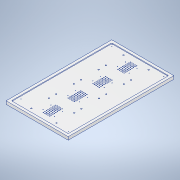
# Autodesk Inventor part: Tamale Assembly Plate
Saved by Autodesk Inventor 2022 (Build 260153000, 153)
## iProperties
Created: 2021-07-29
Part Number: Tamale Assembly Plate
Material: Aluminum 6061
Document SubType Name: Modeling
Designer: Caleb
Density: 2.7 g/cm^3
Appearance: Aluminum - Flat
Author: Caleb
Autodesk Inventor part; units mm, degrees
ref_plane "YZ Plane" through (0, 0, 0) normal (1, 0, 0) x (0, 1, 0)
ref_plane "XZ Plane" through (0, 0, 0) normal (0, 1, 0) x (-1, 0, 0)
ref_plane "XY Plane" through (0, 0, 0) normal (0, 0, 1) x (1, 0, 0)
sketch "Sketch1" plane through (0, 0, 0) normal (0, 1, 0) x (-1, 0, 0)
  line L0 (-63.5, -107.95) -> (63.5, -107.95)
  line L1 (63.5, -107.95) -> (63.5, 107.95)
  line L2 (63.5, 107.95) -> (-63.5, 107.95)
  line L3 (-63.5, 107.95) -> (-63.5, -107.95)
  line L4 (-63.5, -107.95) -> (63.5, 107.95) construction
  line L5 (63.5, -107.95) -> (-63.5, 107.95) construction
  point P0 (0, 0)
  dimension "d0" = 127
  dimension "d1" = 215.9
  constraints: 12 end point, 2 midpoint, 2 parallel, 1 horizontal, 1 perpendicular
  measures "d0" distance of L2.end L1.end
  measures "d1" distance of L0.end L1.end
extrude "Extrusion1" add sketch "Sketch1" along normal blind 6.35
sketch "Sketch2" plane through (0, 6.35, 0) normal (0, 1, 0) x (1, 0, 0)
  line L0 (56.15, 102.6) -> (-56.15, 102.6)
  line L1 (-58.15, 100.6) -> (-58.15, -100.6)
  line L2 (-56.15, -102.6) -> (56.15, -102.6)
  line L3 (58.15, -100.6) -> (58.15, 100.6)
  line L4 (58.15, 102.6) -> (-58.15, -102.6) construction
  line L5 (-58.15, 102.6) -> (58.15, -102.6) construction
  line L6 (-63.5, -107.95) -> (63.5, -107.95) projected
  line L7 (-63.5, 107.95) -> (-63.5, -107.95) projected
  line L8 (63.5, 107.95) -> (-63.5, 107.95) projected
  line L9 (63.5, -107.95) -> (63.5, 107.95) projected
  arc A0 (-58.15, -100.6) -> (-56.15, -102.6) centre (-56.15, -100.6) ccw
  arc A1 (56.15, -102.6) -> (58.15, -100.6) centre (56.15, -100.6) ccw
  arc A2 (58.15, 100.6) -> (56.15, 102.6) centre (56.15, 100.6) ccw
  arc A3 (-56.15, 102.6) -> (-58.15, 100.6) centre (-56.15, 100.6) ccw
  point P0 (0, 0)
  dimension "d4" = 5.35
  dimension "d5" = 5.35
  dimension "d6" = 5.35
  dimension "d77" = 2
  constraints: 12 end point, 8 point on circle, 8 point on line, 8 tangent, 4 centre point, 3 equal radius, 2 midpoint, 2 parallel, 1 horizontal, 1 perpendicular
  measures "d4" distance between parallel lines of L2 L6
  measures "d5" distance between parallel lines of L0 L8
  measures "d6" distance between parallel lines of L7 L1
  measures "d77" radius of A0
extrude "Extrusion2" cut sketch "Sketch2" against normal blind 1.6 contours A2 L3 A1 L2 A0 L1 A3 L0
sketch "Sketch3" plane through (0, 4.75, 0) normal (0, 1, 0) x (1, 0, 0)
  line L0 (-58.15, -100.6) -> (-58.15, 100.6) projected
  line L1 (56.15, -102.6) -> (-56.15, -102.6) projected
  point P0 (0, 0)
  point P1 (-25.75, -94.25)
  point P2 (-25.75, -58.15)
  point P3 (25.75, -94.25)
  point P4 (25.75, -58.15)
  point P5 (-57.15, -101.6)
  point P6 (-57.15, 101.6)
  point P7 (57.15, -101.6)
  point P8 (-25.75, -43.45)
  point P9 (25.75, -43.45)
  point P10 (25.75, -7.35)
  point P11 (-25.75, -7.35)
  point P12 (-25.75, 7.35)
  point P13 (25.75, 7.35)
  point P14 (25.75, 43.45)
  point P15 (-25.75, 43.45)
  point P16 (-25.75, 58.15)
  point P17 (25.75, 58.15)
  point P18 (25.75, 94.25)
  point P19 (-25.75, 94.25)
  dimension "d9" = 32.4
  dimension "d10" = 8.35
  dimension "d11" = 36.1
  dimension "d12" = 51.5
  dimension "d15" = 50.8
  constraints: 14 vertical alignment, 2 horizontal alignment, 2 other
  measures "d11" distance of point (-25.75, -58.15) point (-25.75, -94.25)
  measures "d12" distance of point (25.75, -58.15) point (-25.75, -58.15)
  measures "d15" distance of point (-25.75, -94.25) point (-25.75, -43.45)
hole "Hole1" at (-25.75, 4.75, 94.25) at (-25.75, 4.75, 58.15) at (25.75, 4.75, 94.25) at (25.75, 4.75, 58.15) at (-25.75, 4.75, 43.45) at (25.75, 4.75, 43.45) at (25.75, 4.75, 7.35) at (-25.75, 4.75, 7.35) at (-25.75, 4.75, -7.35) at (25.75, 4.75, -7.35) at (25.75, 4.75, -43.45) at (-25.75, 4.75, -43.45) at (-25.75, 4.75, -58.15) at (25.75, 4.75, -58.15) at (25.75, 4.75, -94.25) at (-25.75, 4.75, -94.25) direction (0, -1, 0) diameter 2.5 end through all
sketch "Sketch4" plane through (0, 4.75, 0) normal (0, 1, 0) x (1, 0, 0)
  line L0 (-58.15, -100.6) -> (-58.15, 100.6) projected
  line L1 (56.15, -102.6) -> (-56.15, -102.6) projected
  line L2 (58.15, 100.6) -> (58.15, -100.6) projected
  line L3 (-56.15, 102.6) -> (56.15, 102.6) projected
  point P0 (0, 0)
  point P1 (-53.15, -87.9)
  point P2 (-57.15, -101.6)
  point P3 (-57.15, 101.6)
  point P4 (57.15, -101.6)
  point P5 (53.15, -97.6)
  point P6 (53.15, 97.6)
  point P7 (-53.15, 97.6)
  point P8 (57.15, 101.6)
  point P9 (-11.765, -84.2)
  point P10 (-11.765, -68.2)
  point P11 (11.766, -84.2)
  point P12 (11.766, -68.2)
  point P13 (-11.765, -33.4)
  point P14 (-11.765, -17.4)
  point P15 (11.766, -17.4)
  point P16 (11.766, -33.4)
  point P17 (-11.765, 17.4)
  point P18 (-11.765, 33.4)
  point P19 (11.766, 33.4)
  point P20 (11.766, 17.4)
  point P21 (-11.765, 68.2)
  point P22 (-11.765, 84.2)
  point P23 (11.766, 84.2)
  point P24 (11.766, 68.2)
  point P25 (58.15, -100.6)
  dimension "d27" = 5
  dimension "d28" = 14.7
  dimension "d29" = 5
  dimension "d30" = 5
  dimension "d31" = 5
  dimension "d32" = 5
  dimension "d33" = 5
  dimension "d34" = 5
  dimension "d35" = 46.385
  dimension "d36" = 18.4
  dimension "d37" = 16
  dimension "d38" = 23.531
  dimension "d41" = 50.8
  constraints: 14 vertical alignment, 2 horizontal alignment, 4 other
  measures "d37" distance of point (-11.765, -68.2) point (-11.765, -84.2)
  measures "d38" distance of point (11.766, -84.2) point (-11.765, -84.2)
  measures "d41" distance of point (-11.765, -84.2) point (-11.765, -33.4)
hole "Hole2" at (-53.15, 4.75, 87.9) at (53.15, 4.75, 97.6) at (53.15, 4.75, -97.6) at (-53.15, 4.75, -97.6) at (-11.765, 4.75, 84.2) at (-11.765, 4.75, 68.2) at (11.766, 4.75, 84.2) at (11.766, 4.75, 68.2) at (-11.765, 4.75, 33.4) at (-11.765, 4.75, 17.4) at (11.766, 4.75, 17.4) at (11.766, 4.75, 33.4) at (-11.765, 4.75, -17.4) at (-11.765, 4.75, -33.4) at (11.766, 4.75, -33.4) at (11.766, 4.75, -17.4) at (-11.765, 4.75, -68.2) at (-11.765, 4.75, -84.2) at (11.766, 4.75, -84.2) at (11.766, 4.75, -68.2) direction (0, -1, 0) diameter 1.0211 end through all thread size "00-96 NS" class "2B" standard "ANSI Unified Screw Threads"
sketch "Sketch5" plane through (0, 4.75, 0) normal (0, 1, 0) x (1, 0, 0)
  line L0 (56.15, -102.6) -> (-56.15, -102.6) projected
  line L1 (-58.15, -100.6) -> (-58.15, 100.6) projected
  point P0 (0, 0)
  point P1 (-6.35, -88.9)
  point P2 (57.15, -101.6)
  point P3 (-57.15, -101.6)
  point P4 (-57.15, 101.6)
  point P5 (-6.35, -85.725)
  point P6 (-6.35, -82.55)
  point P7 (-6.35, -79.375)
  point P8 (-6.35, -76.2)
  point P9 (-6.35, -73.025)
  point P10 (-6.35, -69.85)
  point P11 (-6.35, -66.675)
  point P12 (-6.35, -63.5)
  point P13 (-3.175, -88.9)
  point P14 (-3.175, -85.725)
  point P15 (-3.175, -82.55)
  point P16 (-3.175, -79.375)
  point P17 (-3.175, -76.2)
  point P18 (-3.175, -73.025)
  point P19 (-3.175, -69.85)
  point P20 (-3.175, -66.675)
  point P21 (-3.175, -63.5)
  point P22 (0, -88.9)
  point P23 (0, -85.725)
  point P24 (0, -82.55)
  point P25 (0, -79.375)
  point P26 (0, -76.2)
  point P27 (0, -73.025)
  point P28 (0, -69.85)
  point P29 (0, -66.675)
  point P30 (0, -63.5)
  point P31 (3.175, -88.9)
  point P32 (3.175, -85.725)
  point P33 (3.175, -82.55)
  point P34 (3.175, -79.375)
  point P35 (3.175, -76.2)
  point P36 (3.175, -73.025)
  point P37 (3.175, -69.85)
  point P38 (3.175, -66.675)
  point P39 (3.175, -63.5)
  point P40 (6.35, -88.9)
  point P41 (6.35, -85.725)
  point P42 (6.35, -82.55)
  point P43 (6.35, -79.375)
  point P44 (6.35, -76.2)
  point P45 (6.35, -73.025)
  point P46 (6.35, -69.85)
  point P47 (6.35, -66.675)
  point P48 (6.35, -63.5)
  point P49 (6.35, -12.7)
  point P50 (6.35, -15.875)
  point P51 (6.35, -19.05)
  point P52 (6.35, -22.225)
  point P53 (6.35, -25.4)
  point P54 (6.35, -28.575)
  point P55 (6.35, -31.75)
  point P56 (6.35, -34.925)
  point P57 (6.35, -38.1)
  point P58 (3.175, -12.7)
  point P59 (3.175, -15.875)
  point P60 (3.175, -19.05)
  point P61 (3.175, -22.225)
  point P62 (3.175, -25.4)
  point P63 (3.175, -28.575)
  point P64 (3.175, -31.75)
  point P65 (3.175, -34.925)
  point P66 (3.175, -38.1)
  point P67 (0, -12.7)
  point P68 (0, -15.875)
  point P69 (0, -19.05)
  point P70 (0, -22.225)
  point P71 (0, -25.4)
  point P72 (0, -28.575)
  point P73 (0, -31.75)
  point P74 (0, -34.925)
  point P75 (0, -38.1)
  point P76 (-3.175, -12.7)
  point P77 (-3.175, -15.875)
  point P78 (-3.175, -19.05)
  point P79 (-3.175, -22.225)
  point P80 (-3.175, -25.4)
  point P81 (-3.175, -28.575)
  point P82 (-3.175, -31.75)
  point P83 (-3.175, -34.925)
  point P84 (-3.175, -38.1)
  point P85 (-6.35, -12.7)
  point P86 (-6.35, -15.875)
  point P87 (-6.35, -19.05)
  point P88 (-6.35, -22.225)
  point P89 (-6.35, -25.4)
  point P90 (-6.35, -28.575)
  point P91 (-6.35, -31.75)
  point P92 (-6.35, -34.925)
  point P93 (-6.35, -38.1)
  point P94 (6.35, 38.1)
  point P95 (6.35, 34.925)
  point P96 (6.35, 31.75)
  point P97 (6.35, 28.575)
  point P98 (6.35, 25.4)
  point P99 (6.35, 22.225)
  point P100 (6.35, 19.05)
  point P101 (6.35, 15.875)
  point P102 (6.35, 12.7)
  point P103 (3.175, 38.1)
  point P104 (3.175, 34.925)
  point P105 (3.175, 31.75)
  point P106 (3.175, 28.575)
  point P107 (3.175, 25.4)
  point P108 (3.175, 22.225)
  point P109 (3.175, 19.05)
  point P110 (3.175, 15.875)
  point P111 (3.175, 12.7)
  point P112 (0, 38.1)
  point P113 (0, 34.925)
  point P114 (0, 31.75)
  point P115 (0, 28.575)
  point P116 (0, 25.4)
  point P117 (0, 22.225)
  point P118 (0, 19.05)
  point P119 (0, 15.875)
  point P120 (0, 12.7)
  point P121 (-3.175, 38.1)
  point P122 (-3.175, 34.925)
  point P123 (-3.175, 31.75)
  point P124 (-3.175, 28.575)
  point P125 (-3.175, 25.4)
  point P126 (-3.175, 22.225)
  point P127 (-3.175, 19.05)
  point P128 (-3.175, 15.875)
  point P129 (-3.175, 12.7)
  point P130 (-6.35, 38.1)
  point P131 (-6.35, 34.925)
  point P132 (-6.35, 31.75)
  point P133 (-6.35, 28.575)
  point P134 (-6.35, 25.4)
  point P135 (-6.35, 22.225)
  point P136 (-6.35, 19.05)
  point P137 (-6.35, 15.875)
  point P138 (-6.35, 12.7)
  point P139 (6.35, 88.9)
  point P140 (6.35, 85.725)
  point P141 (6.35, 82.55)
  point P142 (6.35, 79.375)
  point P143 (6.35, 76.2)
  point P144 (6.35, 73.025)
  point P145 (6.35, 69.85)
  point P146 (6.35, 66.675)
  point P147 (6.35, 63.5)
  point P148 (3.175, 88.9)
  point P149 (3.175, 85.725)
  point P150 (3.175, 82.55)
  point P151 (3.175, 79.375)
  point P152 (3.175, 76.2)
  point P153 (3.175, 73.025)
  point P154 (3.175, 69.85)
  point P155 (3.175, 66.675)
  point P156 (3.175, 63.5)
  point P157 (0, 88.9)
  point P158 (0, 85.725)
  point P159 (0, 82.55)
  point P160 (0, 79.375)
  point P161 (0, 76.2)
  point P162 (0, 73.025)
  point P163 (0, 69.85)
  point P164 (0, 66.675)
  point P165 (0, 63.5)
  point P166 (-3.175, 88.9)
  point P167 (-3.175, 85.725)
  point P168 (-3.175, 82.55)
  point P169 (-3.175, 79.375)
  point P170 (-3.175, 76.2)
  point P171 (-3.175, 73.025)
  point P172 (-3.175, 69.85)
  point P173 (-3.175, 66.675)
  point P174 (-3.175, 63.5)
  point P175 (-6.35, 88.9)
  point P176 (-6.35, 85.725)
  point P177 (-6.35, 82.55)
  point P178 (-6.35, 79.375)
  point P179 (-6.35, 76.2)
  point P180 (-6.35, 73.025)
  point P181 (-6.35, 69.85)
  point P182 (-6.35, 66.675)
  point P183 (-6.35, 63.5)
  dimension "d53" = 13.7
  dimension "d54" = 51.8
  dimension "d57" = 3.175
  dimension "d60" = 3.175
  dimension "d65" = 50.8
  constraints: 143 vertical alignment, 36 horizontal alignment, 2 other
  measures "d57" distance of point (-6.35, -88.9) point (-6.35, -85.725)
  measures "d60" distance of point (-6.35, -88.9) point (-3.175, -88.9)
  measures "d65" distance of point (6.35, -63.5) point (6.35, -12.7)
hole "Hole3" at (-6.35, 4.75, 88.9) at (-6.35, 4.75, 85.725) at (-6.35, 4.75, 82.55) at (-6.35, 4.75, 79.375) at (-6.35, 4.75, 76.2) at (-6.35, 4.75, 73.025) at (-6.35, 4.75, 69.85) at (-6.35, 4.75, 66.675) at (-6.35, 4.75, 63.5) at (-3.175, 4.75, 88.9) at (-3.175, 4.75, 85.725) at (-3.175, 4.75, 82.55) at (-3.175, 4.75, 79.375) at (-3.175, 4.75, 76.2) at (-3.175, 4.75, 73.025) at (-3.175, 4.75, 69.85) at (-3.175, 4.75, 66.675) at (-3.175, 4.75, 63.5) at (0, 4.75, 88.9) at (0, 4.75, 85.725) at (0, 4.75, 82.55) at (0, 4.75, 79.375) at (0, 4.75, 76.2) at (0, 4.75, 73.025) at (0, 4.75, 69.85) at (0, 4.75, 66.675) at (0, 4.75, 63.5) at (3.175, 4.75, 88.9) at (3.175, 4.75, 85.725) at (3.175, 4.75, 82.55) at (3.175, 4.75, 79.375) at (3.175, 4.75, 76.2) at (3.175, 4.75, 73.025) at (3.175, 4.75, 69.85) at (3.175, 4.75, 66.675) at (3.175, 4.75, 63.5) at (6.35, 4.75, 88.9) at (6.35, 4.75, 85.725) at (6.35, 4.75, 82.55) at (6.35, 4.75, 79.375) at (6.35, 4.75, 76.2) at (6.35, 4.75, 73.025) at (6.35, 4.75, 69.85) at (6.35, 4.75, 66.675) at (6.35, 4.75, 63.5) at (6.35, 4.75, 12.7) at (6.35, 4.75, 15.875) at (6.35, 4.75, 19.05) at (6.35, 4.75, 22.225) at (6.35, 4.75, 25.4) direction (0, -1, 0) diameter 1.6 end through all and at (6.35, 4.75, 28.575) (6.35, 4.75, 31.75) (6.35, 4.75, 34.925) (6.35, 4.75, 38.1) (3.175, 4.75, 12.7) (3.175, 4.75, 15.875) (3.175, 4.75, 19.05) (3.175, 4.75, 22.225) (3.175, 4.75, 25.4) (3.175, 4.75, 28.575) (3.175, 4.75, 31.75) (3.175, 4.75, 34.925) (3.175, 4.75, 38.1) (0, 4.75, 12.7) (0, 4.75, 15.875) (0, 4.75, 19.05) (0, 4.75, 22.225) (0, 4.75, 25.4) (0, 4.75, 28.575) (0, 4.75, 31.75) (0, 4.75, 34.925) (0, 4.75, 38.1) (-3.175, 4.75, 12.7) (-3.175, 4.75, 15.875) (-3.175, 4.75, 19.05) (-3.175, 4.75, 22.225) (-3.175, 4.75, 25.4) (-3.175, 4.75, 28.575) (-3.175, 4.75, 31.75) (-3.175, 4.75, 34.925) (-3.175, 4.75, 38.1) (-6.35, 4.75, 12.7) (-6.35, 4.75, 15.875) (-6.35, 4.75, 19.05) (-6.35, 4.75, 22.225) (-6.35, 4.75, 25.4) (-6.35, 4.75, 28.575) (-6.35, 4.75, 31.75) (-6.35, 4.75, 34.925) (-6.35, 4.75, 38.1) (6.35, 4.75, -38.1) (6.35, 4.75, -34.925) (6.35, 4.75, -31.75) (6.35, 4.75, -28.575) (6.35, 4.75, -25.4) (6.35, 4.75, -22.225) (6.35, 4.75, -19.05) (6.35, 4.75, -15.875) (6.35, 4.75, -12.7) (3.175, 4.75, -38.1) (3.175, 4.75, -34.925) (3.175, 4.75, -31.75) (3.175, 4.75, -28.575) (3.175, 4.75, -25.4) (3.175, 4.75, -22.225) (3.175, 4.75, -19.05) (3.175, 4.75, -15.875) (3.175, 4.75, -12.7) (0, 4.75, -38.1) (0, 4.75, -34.925) (0, 4.75, -31.75) (0, 4.75, -28.575) (0, 4.75, -25.4) (0, 4.75, -22.225) (0, 4.75, -19.05) (0, 4.75, -15.875) (0, 4.75, -12.7) (-3.175, 4.75, -38.1) (-3.175, 4.75, -34.925) (-3.175, 4.75, -31.75) (-3.175, 4.75, -28.575) (-3.175, 4.75, -25.4) (-3.175, 4.75, -22.225) (-3.175, 4.75, -19.05) (-3.175, 4.75, -15.875) (-3.175, 4.75, -12.7) (-6.35, 4.75, -38.1) (-6.35, 4.75, -34.925) (-6.35, 4.75, -31.75) (-6.35, 4.75, -28.575) (-6.35, 4.75, -25.4) (-6.35, 4.75, -22.225) (-6.35, 4.75, -19.05) (-6.35, 4.75, -15.875) (-6.35, 4.75, -12.7) (6.35, 4.75, -88.9) (6.35, 4.75, -85.725) (6.35, 4.75, -82.55) (6.35, 4.75, -79.375) (6.35, 4.75, -76.2) (6.35, 4.75, -73.025) (6.35, 4.75, -69.85) (6.35, 4.75, -66.675) (6.35, 4.75, -63.5) (3.175, 4.75, -88.9) (3.175, 4.75, -85.725) (3.175, 4.75, -82.55) (3.175, 4.75, -79.375) (3.175, 4.75, -76.2) (3.175, 4.75, -73.025) (3.175, 4.75, -69.85) (3.175, 4.75, -66.675) (3.175, 4.75, -63.5) (0, 4.75, -88.9) (0, 4.75, -85.725) (0, 4.75, -82.55) (0, 4.75, -79.375) (0, 4.75, -76.2) (0, 4.75, -73.025) (0, 4.75, -69.85) (0, 4.75, -66.675) (0, 4.75, -63.5) (-3.175, 4.75, -88.9) (-3.175, 4.75, -85.725) (-3.175, 4.75, -82.55) (-3.175, 4.75, -79.375) (-3.175, 4.75, -76.2) (-3.175, 4.75, -73.025) (-3.175, 4.75, -69.85) (-3.175, 4.75, -66.675) (-3.175, 4.75, -63.5) (-6.35, 4.75, -88.9) (-6.35, 4.75, -85.725) (-6.35, 4.75, -82.55) (-6.35, 4.75, -79.375) (-6.35, 4.75, -76.2) (-6.35, 4.75, -73.025) (-6.35, 4.75, -69.85) (-6.35, 4.75, -66.675) (-6.35, 4.75, -63.5)
body "Solid1"
